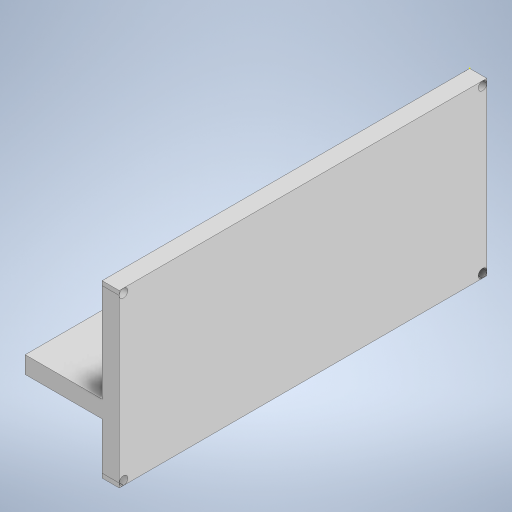
# Autodesk Inventor part: ultrassom
Saved by Autodesk Inventor 2024 (Build 280153020, 153B)
## iProperties
Created: 2023-06-19
Part Number: ultrassom
Material: Genérico
Document SubType Name: Modeling
Designer: victo
Density: 1 g/cm^3
Appearance: Padrão
Author: victo
Autodesk Inventor part; units mm, degrees
ref_plane "YZ Plane" through (0, 0, 0) normal (1, 0, 0) x (0, 1, 0)
ref_plane "XZ Plane" through (0, 0, 0) normal (0, 1, 0) x (-1, 0, 0)
ref_plane "XY Plane" through (0, 0, 0) normal (0, 0, 1) x (1, 0, 0)
sketch "Esboço1" plane through (0, 0, 0) normal (1, 0, 0) x (0, 1, 0)
  line L0 (0, 0) -> (0, 43)
  line L1 (0, 43) -> (20, 43)
  line L2 (20, 43) -> (20, 0)
  line L3 (20, 0) -> (0, 0)
  dimension "d0" = 43
  dimension "d1" = 20
  constraints: 8 end point, 3 perpendicular, 1 vertical
  measures "d0" distance of L0.start L0.end
  measures "d1" distance of L0.end L1.end
extrude "Extrusão1" add sketch "Esboço1" along normal blind 2
sketch "Esboço2" plane through (2, 0, 0) normal (1, 0, 0) x (0, 0, -1)
  line L0 (-43, 20) -> (-43, 0) projected
  line L1 (-43, 0) -> (0, 0) projected
  circle A0 centre (-0.5, 0.4996) radius 0.5
  circle A1 centre (-0.5, 19.4996) radius 0.5
  circle A2 centre (-42.5, 19.4996) radius 0.5
  circle A3 centre (-42.5, 0.4996) radius 0.5
  point P0 (-42.4796, 0)
  point P1 (-42.5204, 0)
  dimension "d12" = 1
  dimension "d13" = 1
  dimension "d14" = 1
  dimension "d15" = 1
  constraints: 4 centre point
  measures "d12" diameter of A0
  measures "d13" diameter of A1
  measures "d14" diameter of A2
  measures "d15" diameter of A3
extrude "Extrusão2" cut sketch "Esboço2" against normal through all contours A0 | A3 | A2 | A1
sketch "Esboço6" plane through (0, 20, 0) normal (-1, 0, 0) x (0, 0, 1)
  line L0 (0, 0) -> (43, 0) projected
  line L1 (11.5781, -12) -> (0, -12)
  line L2 (0, -19.5004) -> (0, -0.5004) projected
  line L3 (11.5781, -14) -> (0, -14)
  line L4 (0, -12) -> (0, -14)
  line L5 (11.5781, -12) -> (43, -12)
  line L6 (43, -12) -> (43, -14)
  line L7 (43, -0.5004) -> (43, -19.5004) projected
  line L8 (11.5781, -14) -> (43, -14)
  point P0 (0, -20)
  dimension "d36" = 2
  constraints: 12 end point, 3 point on line, 2 horizontal, 1 collinear, 1 perpendicular
  measures "d36" distance of L1.start L3.start
extrude "Extrusão5" add sketch "Esboço6" along normal blind 9
sketch "Esboço8" plane through (0, 8, 43) normal (0, 1, 0) x (1, 0, 0)
  line L0 (-9, 0) -> (-9, 43) projected
  line L1 (0, 43) -> (-9, 43) projected
  line L2 (0, 43) -> (0, 0) projected
  circle A0 centre (-4.4997, 32.2499) radius 1.5
  circle A1 centre (-4.4997, 21.5) radius 1.5
  circle A2 centre (-4.4997, 10.7499) radius 1.5
  dimension "d53" = 3
  dimension "d54" = 3
  dimension "d55" = 3
  constraints: 3 centre point
  measures "d53" diameter of A0
  measures "d54" diameter of A1
  measures "d55" diameter of A2
sketch "Esboço9" plane through (0, 20, 43) normal (0, 1, 0) x (1, 0, 0)
  point P0 (0, 43)
extrude "Extrusão7" cut sketch "Esboço8" against normal up to next
